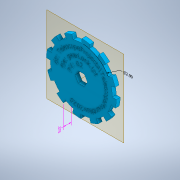
# Autodesk Inventor part: gearLockTopHalf
Saved by Autodesk Inventor 2021.2 (Build 252289000, 289)
## iProperties
Created: 2020-11-07
Part Number: gearLockTopHalf
Material: PC/ABS Plastic
Document SubType Name: Modeling
Designer: robst
Density: 0.357273 g/cm^3
Appearance: Sky Blue Medium
Author: robst
Autodesk Inventor part; units mm, degrees
(part 1 of 2)
ref_plane "YZ Plane" through (0, 0, 0) normal (1, 0, 0) x (0, 1, 0)
ref_plane "XZ Plane" through (0, 0, 0) normal (0, 1, 0) x (-1, 0, 0)
sketch "Sketch1" plane through (0, 0, 0) normal (0, 0, 1) x (1, 0, 0)
  circle A0 centre (0, 0) radius 37.9095
  dimension "d0" = 75.819
  constraints: 1 centre point, 1 coincident
  measures "d0" diameter of A0
extrude "Extrusion1" add sketch "Sketch1" along normal mid plane 9.525
sketch "Sketch10" plane through (0, 0, 4.7625) normal (0, 0, 1) x (1, 0, 0)
  line L0 (7.5523, 0) -> (3.7762, -6.5405)
  line L1 (3.7762, -6.5405) -> (-3.7762, -6.5405)
  line L2 (-3.7762, -6.5405) -> (-7.5523, 0)
  line L3 (-7.5523, 0) -> (-3.7762, 6.5405)
  line L4 (-3.7762, 6.5405) -> (3.7762, 6.5405)
  line L5 (3.7762, 6.5405) -> (7.5523, 0)
  point P0 (0, 0)
  point P1 (0, 0)
  dimension "d55" = 13.081
  constraints: 12 end point, 1 coincident, 1 horizontal, 13 other
  measures "d55" distance between parallel lines of L1 L4
extrude "Extrusion11" cut sketch "Sketch10" against normal through all
sketch "Sketch17" plane through (0, 0, 4.7625) normal (0, 0, 1) x (1, 0, 0)
  circle A0 centre (0, 0) radius 37.9095 projected
  arc A1 (9.4918, 36.702) -> (0, 37.9095) centre (0, 0) ccw
  arc A2 (10.6984, 41.5413) -> (0, 42.8968) centre (0, 0) ccw
  line L0 (0, 0) -> (0, 42.8968) construction
  line L1 (0, 0) -> (0.7487, 42.8902)
  line L2 (9.4918, 36.702) -> (10.6984, 41.5413)
  point P0 (0.6616, 37.9037)
  dimension "d123" = 4.9873
  dimension "d124" = 1
  dimension "d125" = 13
  dimension "d131" = 75.819
  dimension "d132" = 85.7936
  constraints: 6 end point, 5 point on circle, 2 centre point, 2 coincident, 1 concentric, 1 point on line, 1 vertical
  measures "d123" radial gap between concentric circles of A2 A0
  measures "d124" angle of L1 L0
  measures "d125" angle of L2 L1
  measures "d131" diameter of A0
  measures "d132" diameter of A2
extrude "Extrusion19" add sketch "Sketch17" against normal blind 9.525 contours A0 L1 A2 L2
pattern_circular "Circular Pattern11" count 12 over 360 about axis through (0, 0, -10) along (0, 0, 1) of "Extrusion19"
sketch "Sketch28" plane through (0, 0, 4.7625) normal (0, 0, 1) x (1, 0, 0)
  circle A0 centre (0, 0) radius 28.575 construction
  line L0 (-28.4112, 3.3885) -> (-28.4545, 2.7478)
  line L1 (-28.4545, 2.7478) -> (-28.8406, 2.7739)
  spline S0 degree 2 poles (-28.8406, 2.7739) (-28.7274, 2.6177) (-28.5778, 2.3889) (-28.5179, 2.2363) knots 0 0 0 1 2 2 2
  spline S1 degree 2 poles (-28.5179, 2.2363) (-28.4614, 2.0963) (-28.4113, 1.8) (-28.4243, 1.607) knots 0 0 0 1 2 2 2
  spline S2 degree 2 poles (-28.4243, 1.607) (-28.4454, 1.2948) (-28.7397, 0.7866) (-29.0027, 0.6187) knots 0 0 0 1 2 2 2
  spline S3 degree 2 poles (-29.0027, 0.6187) (-29.2657, 0.4508) (-30.0189, 0.2953) (-30.4995, 0.3278) knots 0 0 0 1 2 2 2
  spline S4 degree 2 poles (-30.4995, 0.3278) (-31.0006, 0.3617) (-31.7142, 0.6698) (-31.9741, 0.9143) knots 0 0 0 1 2 2 2
  spline S5 degree 2 poles (-31.9741, 0.9143) (-32.2064, 1.1404) (-32.4501, 1.7469) (-32.4282, 2.0714) knots 0 0 0 1 2 2 2
  spline S6 degree 2 poles (-32.4282, 2.0714) (-32.4091, 2.3548) (-32.2532, 2.7693) (-32.1059, 2.9945) knots 0 0 0 1 2 2 2
  line L2 (-32.1059, 2.9945) -> (-33.7488, 3.1055)
  line L3 (-33.7488, 3.1055) -> (-33.7055, 3.7463)
  line L4 (-33.7055, 3.7463) -> (-28.4112, 3.3885)
  line L5 (-29.3786, 2.8102) -> (-31.5761, 2.9587)
  spline S7 degree 2 poles (-31.5761, 2.9587) (-31.7072, 2.7283) (-31.8189, 2.3562) (-31.8337, 2.1385) knots 0 0 0 1 2 2 2
  spline S8 degree 2 poles (-31.8337, 2.1385) (-31.867, 1.6456) (-31.1654, 1.0371) (-30.4671, 0.9899) knots 0 0 0 1 2 2 2
  spline S9 degree 2 poles (-30.4671, 0.9899) (-29.7935, 0.9444) (-29.0541, 1.3236) (-29.0222, 1.7959) knots 0 0 0 1 2 2 2
  spline S10 degree 2 poles (-29.0222, 1.7959) (-29.0053, 2.0464) (-29.2009, 2.5713) (-29.3786, 2.8102) knots 0 0 0 1 2 2 2
  line L6 (-28.1448, 4.9503) -> (-28.2489, 4.3166)
  line L7 (-28.2489, 4.3166) -> (-32.0105, 4.9348)
  line L8 (-32.0105, 4.9348) -> (-31.9064, 5.5685)
  line L9 (-31.9064, 5.5685) -> (-28.1448, 4.9503)
  line L10 (-32.5246, 5.7159) -> (-32.6428, 4.9969)
  line L11 (-32.6428, 4.9969) -> (-33.3008, 5.1051)
  line L12 (-33.3008, 5.1051) -> (-33.1827, 5.8241)
  line L13 (-33.1827, 5.8241) -> (-32.5246, 5.7159)
  line L14 (-30.5438, 8.57) -> (-30.5514, 8.538)
  spline S11 degree 2 poles (-30.5514, 8.538) (-30.5887, 8.4707) (-30.6341, 8.3165) (-30.6599, 8.2084) knots 0 0 0 1 2 2 2
  spline S12 degree 2 poles (-30.6599, 8.2084) (-30.7203, 7.9562) (-30.6189, 7.407) (-30.4563, 7.1311) knots 0 0 0 1 2 2 2
  line L15 (-30.4563, 7.1311) -> (-27.8259, 6.5017)
  line L16 (-27.8259, 6.5017) -> (-27.9754, 5.8771)
  line L17 (-27.9754, 5.8771) -> (-31.6828, 6.7642)
  line L18 (-31.6828, 6.7642) -> (-31.5333, 7.3888)
  line L19 (-31.5333, 7.3888) -> (-30.9808, 7.2566)
  spline S13 degree 2 poles (-30.9808, 7.2566) (-31.2037, 7.6697) (-31.3302, 8.2376) (-31.2727, 8.4778) knots 0 0 0 1 2 2 2
  spline S14 degree 2 poles (-31.2727, 8.4778) (-31.2497, 8.5739) (-31.2187, 8.6681) (-31.1924, 8.7252) knots 0 0 0 1 2 2 2
  line L20 (-31.1924, 8.7252) -> (-30.5438, 8.57)
  line L21 (-26.9763, 9.4327) -> (-27.2343, 8.6595)
  line L22 (-27.2343, 8.6595) -> (-28.1559, 8.9671)
  line L23 (-28.1559, 8.9671) -> (-27.8979, 9.7403)
  line L24 (-27.8979, 9.7403) -> (-26.9763, 9.4327)
  line L25 (-29.6707, 10.332) -> (-29.9288, 9.5588)
  line L26 (-29.9288, 9.5588) -> (-30.8503, 9.8663)
  line L27 (-30.8503, 9.8663) -> (-30.5923, 10.6395)
  line L28 (-30.5923, 10.6395) -> (-29.6707, 10.332)
  line L29 (-25.0649, 13.7258) -> (-28.9674, 15.9239)
  line L30 (-28.9674, 15.9239) -> (-29.8038, 14.4389)
  line L31 (-29.8038, 14.4389) -> (-30.3275, 14.7339)
  line L32 (-30.3275, 14.7339) -> (-28.3233, 18.2921)
  line L33 (-28.3233, 18.2921) -> (-27.7997, 17.9971)
  line L34 (-27.7997, 17.9971) -> (-28.6361, 16.5121)
  line L35 (-28.6361, 16.5121) -> (-24.7336, 14.314)
  line L36 (-24.7336, 14.314) -> (-25.0649, 13.7258)
  spline S15 degree 2 poles (-22.5342, 17.4324) (-23.0862, 16.7041) (-24.5098, 16.5227) (-25.2644, 17.0946) knots 0 0 0 1 2 2 2
  spline S16 degree 2 poles (-25.2644, 17.0946) (-26.0059, 17.6565) (-26.2959, 19.1005) (-25.8209, 19.7272) knots 0 0 0 1 2 2 2
  spline S17 degree 2 poles (-25.8209, 19.7272) (-25.6071, 20.0093) (-25.1123, 20.3213) (-24.8166, 20.3503) knots 0 0 0 1 2 2 2
  spline S18 degree 2 poles (-24.8166, 20.3503) (-24.5184, 20.3826) (-23.8846, 20.176) (-23.5205, 19.9) knots 0 0 0 1 2 2 2
  line L37 (-23.5205, 19.9) -> (-23.2416, 19.6887)
  line L38 (-23.2416, 19.6887) -> (-24.8355, 17.5856)
  spline S19 degree 2 poles (-24.8355, 17.5856) (-24.3072, 17.1853) (-23.3434, 17.2916) (-22.9853, 17.764) knots 0 0 0 1 2 2 2
  spline S20 degree 2 poles (-22.9853, 17.764) (-22.8585, 17.9313) (-22.6878, 18.3133) (-22.6474, 18.4893) knots 0 0 0 1 2 2 2
  spline S21 degree 2 poles (-22.6474, 18.4893) (-22.6086, 18.6769) (-22.5792, 18.9542) (-22.5844, 19.0563) knots 0 0 0 1 2 2 2
  line L39 (-22.5844, 19.0563) -> (-22.5621, 19.0858)
  line L40 (-22.5621, 19.0858) -> (-22.0043, 18.6631)
  spline S22 degree 2 poles (-22.0043, 18.6631) (-22.0354, 18.5472) (-22.1343, 18.1986) (-22.1843, 18.0712) knots 0 0 0 1 2 2 2
  spline S23 degree 2 poles (-22.1843, 18.0712) (-22.2536, 17.8912) (-22.3949, 17.6161) (-22.5342, 17.4324) knots 0 0 0 1 2 2 2
  spline S24 degree 2 poles (-24.01, 19.4859) (-24.2216, 19.636) (-24.5881, 19.7794) (-24.752, 19.7745) knots 0 0 0 1 2 2 2
  spline S25 degree 2 poles (-24.752, 19.7745) (-24.934, 19.7729) (-25.2667, 19.586) (-25.4234, 19.3794) knots 0 0 0 1 2 2 2
  spline S26 degree 2 poles (-25.4234, 19.3794) (-25.5775, 19.1759) (-25.6725, 18.7985) (-25.6439, 18.5909) knots 0 0 0 1 2 2 2
  spline S27 degree 2 poles (-25.6439, 18.5909) (-25.6095, 18.384) (-25.407, 18.0446) (-25.2259, 17.8815) knots 0 0 0 1 2 2 2
  line L41 (-25.2259, 17.8815) -> (-24.01, 19.4859)
  line L42 (-20.8713, 19.5198) -> (-21.3046, 19.0459)
  line L43 (-21.3046, 19.0459) -> (-25.2207, 22.6267)
  line L44 (-25.2207, 22.6267) -> (-24.7873, 23.1007)
  line L45 (-24.7873, 23.1007) -> (-20.8713, 19.5198)
  spline S28 degree 2 poles (-18.9567, 21.2678) (-19.6329, 20.653) (-21.0656, 20.7357) (-21.7026, 21.4362) knots 0 0 0 1 2 2 2
  spline S29 degree 2 poles (-21.7026, 21.4362) (-22.3285, 22.1246) (-22.3489, 23.5973) (-21.7671, 24.1262) knots 0 0 0 1 2 2 2
  spline S30 degree 2 poles (-21.7671, 24.1262) (-21.5052, 24.3644) (-20.9616, 24.5804) (-20.6656, 24.5547) knots 0 0 0 1 2 2 2
  spline S31 degree 2 poles (-20.6656, 24.5547) (-20.3665, 24.5318) (-19.7813, 24.2125) (-19.4739, 23.8744) knots 0 0 0 1 2 2 2
  line L46 (-19.4739, 23.8744) -> (-19.2385, 23.6155)
  line L47 (-19.2385, 23.6155) -> (-21.1909, 21.8403)
  spline S32 degree 2 poles (-21.1909, 21.8403) (-20.745, 21.3499) (-19.778, 21.2777) (-19.3394, 21.6765) knots 0 0 0 1 2 2 2
  spline S33 degree 2 poles (-19.3394, 21.6765) (-19.1841, 21.8178) (-18.9462, 22.162) (-18.8743, 22.3276) knots 0 0 0 1 2 2 2
  spline S34 degree 2 poles (-18.8743, 22.3276) (-18.8017, 22.5049) (-18.722, 22.7721) (-18.7084, 22.8734) knots 0 0 0 1 2 2 2
  line L48 (-18.7084, 22.8734) -> (-18.681, 22.8984)
  line L49 (-18.681, 22.8984) -> (-18.2102, 22.3806)
  spline S35 degree 2 poles (-18.2102, 22.3806) (-18.262, 22.2723) (-18.4231, 21.9477) (-18.4957, 21.8317) knots 0 0 0 1 2 2 2
  spline S36 degree 2 poles (-18.4957, 21.8317) (-18.5967, 21.6675) (-18.7861, 21.4229) (-18.9567, 21.2678) knots 0 0 0 1 2 2 2
  spline S37 degree 2 poles (-20.031, 23.557) (-20.2116, 23.7434) (-20.5456, 23.9516) (-20.7076, 23.9768) knots 0 0 0 1 2 2 2
  spline S38 degree 2 poles (-20.7076, 23.9768) (-20.8868, 24.0086) (-21.2481, 23.8859) (-21.44, 23.7114) knots 0 0 0 1 2 2 2
  spline S39 degree 2 poles (-21.44, 23.7114) (-21.6289, 23.5397) (-21.7914, 23.1861) (-21.8013, 22.9767) knots 0 0 0 1 2 2 2
  spline S40 degree 2 poles (-21.8013, 22.9767) (-21.8055, 22.7671) (-21.6686, 22.3963) (-21.5205, 22.2028) knots 0 0 0 1 2 2 2
  line L50 (-21.5205, 22.2028) -> (-20.031, 23.557)
  spline S41 degree 2 poles (-16.5837, 23.1592) (-16.8954, 22.937) (-17.5546, 22.72) (-17.7992, 22.6872) knots 0 0 0 1 2 2 2
  line L51 (-17.7992, 22.6872) -> (-18.2173, 23.2739)
  line L52 (-18.2173, 23.2739) -> (-18.1905, 23.293)
  spline S42 degree 2 poles (-18.1905, 23.293) (-18.0852, 23.2872) (-17.8134, 23.2888) (-17.6124, 23.3259) knots 0 0 0 1 2 2 2
  spline S43 degree 2 poles (-17.6124, 23.3259) (-17.4362, 23.3554) (-17.0475, 23.4909) (-16.8765, 23.6127) knots 0 0 0 1 2 2 2
  spline S44 degree 2 poles (-16.8765, 23.6127) (-16.7525, 23.7011) (-16.5081, 23.9612) (-16.4745, 24.0559) knots 0 0 0 1 2 2 2
  spline S45 degree 2 poles (-16.4745, 24.0559) (-16.4227, 24.1889) (-16.4383, 24.3952) (-16.5434, 24.5427) knots 0 0 0 1 2 2 2
  spline S46 degree 2 poles (-16.5434, 24.5427) (-16.6748, 24.7271) (-17.0122, 24.7748) (-17.3157, 24.6545) knots 0 0 0 1 2 2 2
  spline S47 degree 2 poles (-17.3157, 24.6545) (-17.433, 24.6063) (-17.8026, 24.444) (-17.9663, 24.3829) knots 0 0 0 1 2 2 2
  spline S48 degree 2 poles (-17.9663, 24.3829) (-18.3958, 24.2336) (-19.0234, 24.4333) (-19.2408, 24.7384) knots 0 0 0 1 2 2 2
  spline S49 degree 2 poles (-19.2408, 24.7384) (-19.5419, 25.1608) (-19.2834, 26.1387) (-18.7604, 26.5114) knots 0 0 0 1 2 2 2
  spline S50 degree 2 poles (-18.7604, 26.5114) (-18.5023, 26.6954) (-17.8885, 26.9407) (-17.6415, 26.9701) knots 0 0 0 1 2 2 2
  line L53 (-17.6415, 26.9701) -> (-17.2425, 26.4103)
  line L54 (-17.2425, 26.4103) -> (-17.2693, 26.3912)
  spline S51 degree 2 poles (-17.2693, 26.3912) (-17.5852, 26.4087) (-18.206, 26.2443) (-18.4575, 26.0651) knots 0 0 0 1 2 2 2
  spline S52 degree 2 poles (-18.4575, 26.0651) (-18.7156, 25.8811) (-18.9157, 25.4099) (-18.7604, 25.192) knots 0 0 0 1 2 2 2
  spline S53 degree 2 poles (-18.7604, 25.192) (-18.6194, 24.9942) (-18.272, 24.9537) (-17.9943, 25.0606) knots 0 0 0 1 2 2 2
  spline S54 degree 2 poles (-17.9943, 25.0606) (-17.8588, 25.1116) (-17.5275, 25.2568) (-17.3437, 25.3322) knots 0 0 0 1 2 2 2
  spline S55 degree 2 poles (-17.3437, 25.3322) (-16.9396, 25.4887) (-16.3067, 25.3383) (-16.0606, 24.993) knots 0 0 0 1 2 2 2
  spline S56 degree 2 poles (-16.0606, 24.993) (-15.9172, 24.7918) (-15.8215, 24.3242) (-15.8825, 24.0835) knots 0 0 0 1 2 2 2
  spline S57 degree 2 poles (-15.8825, 24.0835) (-15.9489, 23.829) (-16.2652, 23.3862) (-16.5837, 23.1592) knots 0 0 0 1 2 2 2
  spline S58 degree 2 poles (-13.5451, 25.0652) (-13.8904, 24.8728) (-14.5804, 24.7664) (-14.9056, 24.8679) knots 0 0 0 1 2 2 2
  spline S59 degree 2 poles (-14.9056, 24.8679) (-15.2288, 24.9658) (-15.82, 25.4941) (-16.0645, 25.9328) knots 0 0 0 1 2 2 2
  spline S60 degree 2 poles (-16.0645, 25.9328) (-16.309, 26.3715) (-16.4319, 27.1419) (-16.3543, 27.4679) knots 0 0 0 1 2 2 2
  spline S61 degree 2 poles (-16.3543, 27.4679) (-16.2788, 27.7974) (-15.8229, 28.3578) (-15.4849, 28.5462) knots 0 0 0 1 2 2 2
  spline S62 degree 2 poles (-15.4849, 28.5462) (-15.2116, 28.6985) (-14.6147, 28.8284) (-14.3608, 28.8379) knots 0 0 0 1 2 2 2
  line L55 (-14.3608, 28.8379) -> (-14.0102, 28.2086)
  line L56 (-14.0102, 28.2086) -> (-14.0425, 28.1905)
  spline S63 degree 2 poles (-14.0425, 28.1905) (-14.1317, 28.2068) (-14.3909, 28.2321) (-14.562, 28.2263) knots 0 0 0 1 2 2 2
  spline S64 degree 2 poles (-14.562, 28.2263) (-14.7127, 28.2177) (-15.0793, 28.1312) (-15.2231, 28.0511) knots 0 0 0 1 2 2 2
  spline S65 degree 2 poles (-15.2231, 28.0511) (-15.6582, 27.8086) (-15.8202, 26.856) (-15.4855, 26.2554) knots 0 0 0 1 2 2 2
  spline S66 degree 2 poles (-15.4855, 26.2554) (-15.1589, 25.6693) (-14.2816, 25.2957) (-13.8285, 25.5482) knots 0 0 0 1 2 2 2
  spline S67 degree 2 poles (-13.8285, 25.5482) (-13.5552, 25.7005) (-13.1851, 26.2036) (-13.0927, 26.486) knots 0 0 0 1 2 2 2
  line L57 (-13.0927, 26.486) -> (-13.0604, 26.504)
  line L58 (-13.0604, 26.504) -> (-12.7097, 25.8747)
  spline S68 degree 2 poles (-12.7097, 25.8747) (-12.7704, 25.7891) (-12.96, 25.5373) (-13.0466, 25.456) knots 0 0 0 1 2 2 2
  spline S69 degree 2 poles (-13.0466, 25.456) (-13.1664, 25.3327) (-13.3689, 25.1633) (-13.5451, 25.0652) knots 0 0 0 1 2 2 2
  spline S70 degree 2 poles (-9.8925, 28.8813) (-9.53, 27.9888) (-9.9932, 26.6677) (-10.7102, 26.3764) knots 0 0 0 1 2 2 2
  spline S71 degree 2 poles (-10.7102, 26.3764) (-11.4463, 26.0775) (-12.6967, 26.7382) (-13.0468, 27.6002) knots 0 0 0 1 2 2 2
  spline S72 degree 2 poles (-13.0468, 27.6002) (-13.4061, 28.4851) (-12.9346, 29.8185) (-12.2252, 30.1067) knots 0 0 0 1 2 2 2
  spline S73 degree 2 poles (-12.2252, 30.1067) (-11.5081, 30.3979) (-10.2534, 29.77) (-9.8925, 28.8813) knots 0 0 0 1 2 2 2
  spline S74 degree 2 poles (-10.5065, 28.6319) (-10.7854, 29.3184) (-11.5561, 29.783) (-12.0176, 29.5956) knots 0 0 0 1 2 2 2
  spline S75 degree 2 poles (-12.0176, 29.5956) (-12.4791, 29.4081) (-12.7115, 28.5362) (-12.4327, 27.8496) knots 0 0 0 1 2 2 2
  spline S76 degree 2 poles (-12.4327, 27.8496) (-12.1616, 27.1822) (-11.3793, 26.7001) (-10.9178, 26.8875) knots 0 0 0 1 2 2 2
  spline S77 degree 2 poles (-10.9178, 26.8875) (-10.4601, 27.0734) (-10.2308, 27.953) (-10.5065, 28.6319) knots 0 0 0 1 2 2 2
  spline S78 degree 2 poles (-5.9537, 30.0486) (-5.7155, 29.1237) (-6.3152, 27.8045) (-6.9889, 27.631) knots 0 0 0 1 2 2 2
  spline S79 degree 2 poles (-6.9889, 27.631) (-7.264, 27.5601) (-7.7194, 27.5789) (-7.9726, 27.654) knots 0 0 0 1 2 2 2
  line L59 (-7.9726, 27.654) -> (-7.5742, 26.1072)
  line L60 (-7.5742, 26.1072) -> (-8.1961, 25.947)
  line L61 (-8.1961, 25.947) -> (-9.497, 30.998)
  line L62 (-9.497, 30.998) -> (-8.8751, 31.1582)
  line L63 (-8.8751, 31.1582) -> (-8.7755, 30.7715)
  spline S80 degree 2 poles (-8.7755, 30.7715) (-8.5987, 31.0423) (-8.1045, 31.4672) (-7.7736, 31.5524) knots 0 0 0 1 2 2 2
  spline S81 degree 2 poles (-7.7736, 31.5524) (-7.1397, 31.7157) (-6.1714, 30.8938) (-5.9537, 30.0486) knots 0 0 0 1 2 2 2
  spline S82 degree 2 poles (-6.5771, 29.8116) (-6.7403, 30.4454) (-7.3227, 31.0394) (-7.7731, 30.9234) knots 0 0 0 1 2 2 2
  spline S83 degree 2 poles (-7.7731, 30.9234) (-8.0363, 30.8556) (-8.47, 30.4931) (-8.642, 30.2532) knots 0 0 0 1 2 2 2
  line L64 (-8.642, 30.2532) -> (-8.102, 28.1563)
  spline S84 degree 2 poles (-8.102, 28.1563) (-7.829, 28.1033) (-7.4596, 28.1049) (-7.2363, 28.1624) knots 0 0 0 1 2 2 2
  spline S85 degree 2 poles (-7.2363, 28.1624) (-6.754, 28.2866) (-6.4025, 29.1338) (-6.5771, 29.8116) knots 0 0 0 1 2 2 2
  spline S86 degree 2 poles (-3.141, 28.3163) (-4.0483, 28.2065) (-5.1686, 29.1035) (-5.2823, 30.0435) knots 0 0 0 1 2 2 2
  spline S87 degree 2 poles (-5.2823, 30.0435) (-5.3941, 30.9672) (-4.558, 32.1796) (-3.7774, 32.274) knots 0 0 0 1 2 2 2
  spline S88 degree 2 poles (-3.7774, 32.274) (-3.4259, 32.3166) (-2.8576, 32.178) (-2.6311, 31.9856) knots 0 0 0 1 2 2 2
  spline S89 degree 2 poles (-2.6311, 31.9856) (-2.4006, 31.7937) (-2.1084, 31.1946) (-2.0535, 30.7409) knots 0 0 0 1 2 2 2
  line L65 (-2.0535, 30.7409) -> (-2.0115, 30.3936)
  line L66 (-2.0115, 30.3936) -> (-4.6312, 30.0767)
  spline S90 degree 2 poles (-4.6312, 30.0767) (-4.5516, 29.4187) (-3.805, 28.7999) (-3.2165, 28.8711) knots 0 0 0 1 2 2 2
  spline S91 degree 2 poles (-3.2165, 28.8711) (-3.008, 28.8963) (-2.6148, 29.0392) (-2.4602, 29.1326) knots 0 0 0 1 2 2 2
  spline S92 degree 2 poles (-2.4602, 29.1326) (-2.2984, 29.2351) (-2.0787, 29.4068) (-2.009, 29.4816) knots 0 0 0 1 2 2 2
  line L67 (-2.009, 29.4816) -> (-1.9722, 29.486)
  line L68 (-1.9722, 29.486) -> (-1.8881, 28.7913)
  spline S93 degree 2 poles (-1.8881, 28.7913) (-1.9931, 28.733) (-2.3124, 28.5616) (-2.4387, 28.509) knots 0 0 0 1 2 2 2
  spline S94 degree 2 poles (-2.4387, 28.509) (-2.6162, 28.4337) (-2.9122, 28.3439) (-3.141, 28.3163) knots 0 0 0 1 2 2 2
  spline S95 degree 2 poles (-2.6915, 30.8048) (-2.7308, 31.0612) (-2.8826, 31.4244) (-3.0001, 31.5387) knots 0 0 0 1 2 2 2
  spline S96 degree 2 poles (-3.0001, 31.5387) (-3.1277, 31.6684) (-3.4934, 31.7776) (-3.7509, 31.7465) knots 0 0 0 1 2 2 2
  spline S97 degree 2 poles (-3.7509, 31.7465) (-4.0042, 31.7158) (-4.3415, 31.5216) (-4.4708, 31.3567) knots 0 0 0 1 2 2 2
  spline S98 degree 2 poles (-4.4708, 31.3567) (-4.5956, 31.1881) (-4.6987, 30.8066) (-4.69, 30.563) knots 0 0 0 1 2 2 2
  line L69 (-4.69, 30.563) -> (-2.6915, 30.8048)
  spline S99 degree 2 poles (2.1582, 32.1015) (2.1545, 31.7721) (1.9132, 31.182) (1.701, 30.9785) knots 0 0 0 1 2 2 2
  spline S100 degree 2 poles (1.701, 30.9785) (1.4346, 30.7221) (0.7195, 30.4625) (0.1761, 30.4686) knots 0 0 0 1 2 2 2
  line L70 (0.1761, 30.4686) -> (-0.3961, 30.475)
  line L71 (-0.3961, 30.475) -> (-0.4173, 28.5815)
  line L72 (-0.4173, 28.5815) -> (-1.0924, 28.589)
  line L73 (-1.0924, 28.589) -> (-1.0355, 33.6687)
  line L74 (-1.0355, 33.6687) -> (0.2406, 33.6544)
  spline S101 degree 2 poles (0.2406, 33.6544) (0.6934, 33.6494) (1.3256, 33.4941) (1.5666, 33.3226) knots 0 0 0 1 2 2 2
  spline S102 degree 2 poles (1.5666, 33.3226) (1.8485, 33.1259) (2.1629, 32.5255) (2.1582, 32.1015) knots 0 0 0 1 2 2 2
  spline S103 degree 2 poles (1.454, 32.0888) (1.457, 32.3522) (1.2802, 32.7412) (1.0963, 32.8667) knots 0 0 0 1 2 2 2
  spline S104 degree 2 poles (1.0963, 32.8667) (0.937, 32.9756) (0.5098, 33.0668) (0.1929, 33.0703) knots 0 0 0 1 2 2 2
  line L75 (0.1929, 33.0703) -> (-0.367, 33.0766)
  line L76 (-0.367, 33.0766) -> (-0.3896, 31.0513)
  line L77 (-0.3896, 31.0513) -> (0.0714, 31.0462)
  spline S105 degree 2 poles (0.0714, 31.0462) (0.4831, 31.0416) (0.9908, 31.1676) (1.1574, 31.3387) knots 0 0 0 1 2 2 2
  spline S106 degree 2 poles (1.1574, 31.3387) (1.3114, 31.4893) (1.4513, 31.8459) (1.454, 32.0888) knots 0 0 0 1 2 2 2
  line L78 (5.093, 31.3118) -> (5.0603, 31.3158)
  spline S107 degree 2 poles (5.0603, 31.3158) (4.9893, 31.3453) (4.8309, 31.3731) (4.7206, 31.3867) knots 0 0 0 1 2 2 2
  spline S108 degree 2 poles (4.7206, 31.3867) (4.4632, 31.4184) (3.9289, 31.2561) (3.6729, 31.0637) knots 0 0 0 1 2 2 2
  line L79 (3.6729, 31.0637) -> (3.3422, 28.3793)
  line L80 (3.3422, 28.3793) -> (2.7049, 28.4578)
  line L81 (2.7049, 28.4578) -> (3.1709, 32.2412)
  line L82 (3.1709, 32.2412) -> (3.8083, 32.1627)
  line L83 (3.8083, 32.1627) -> (3.7388, 31.5989)
  spline S109 degree 2 poles (3.7388, 31.5989) (4.1244, 31.8666) (4.6745, 32.056) (4.9196, 32.0258) knots 0 0 0 1 2 2 2
  spline S110 degree 2 poles (4.9196, 32.0258) (5.0177, 32.0138) (5.1147, 31.9935) (5.1745, 31.9737) knots 0 0 0 1 2 2 2
  line L84 (5.1745, 31.9737) -> (5.093, 31.3118)
  spline S111 degree 2 poles (8.6902, 29.2655) (8.4679, 28.3282) (7.3244, 27.5205) (6.5714, 27.6991) knots 0 0 0 1 2 2 2
  spline S112 degree 2 poles (6.5714, 27.6991) (5.7983, 27.8825) (5.1629, 29.1459) (5.3776, 30.0512) knots 0 0 0 1 2 2 2
  spline S113 degree 2 poles (5.3776, 30.0512) (5.598, 30.9805) (6.7554, 31.7933) (7.5005, 31.6166) knots 0 0 0 1 2 2 2
  spline S114 degree 2 poles (7.5005, 31.6166) (8.2535, 31.438) (8.9116, 30.1988) (8.6902, 29.2655) knots 0 0 0 1 2 2 2
  spline S115 degree 2 poles (8.0453, 29.4185) (8.2163, 30.1395) (7.8578, 30.9649) (7.3732, 31.0798) knots 0 0 0 1 2 2 2
  spline S116 degree 2 poles (7.3732, 31.0798) (6.8885, 31.1948) (6.1935, 30.6192) (6.0225, 29.8982) knots 0 0 0 1 2 2 2
  spline S117 degree 2 poles (6.0225, 29.8982) (5.8563, 29.1972) (6.214, 28.3508) (6.6987, 28.2359) knots 0 0 0 1 2 2 2
  spline S118 degree 2 poles (6.6987, 28.2359) (7.1793, 28.1219) (7.8762, 28.7055) (8.0453, 29.4185) knots 0 0 0 1 2 2 2
  spline S119 degree 2 poles (9.8099, 26.7294) (9.5969, 26.1148) (8.7119, 25.6982) (8.1324, 25.899) knots 0 0 0 1 2 2 2
  spline S120 degree 2 poles (8.1324, 25.899) (8.0312, 25.934) (7.789, 26.0397) (7.6752, 26.101) knots 0 0 0 1 2 2 2
  line L85 (7.6752, 26.101) -> (7.8638, 26.6456)
  line L86 (7.8638, 26.6456) -> (7.8988, 26.6334)
  spline S121 degree 2 poles (7.8988, 26.6334) (7.9635, 26.5936) (8.1238, 26.5032) (8.2016, 26.4762) knots 0 0 0 1 2 2 2
  spline S122 degree 2 poles (8.2016, 26.4762) (8.4428, 26.3927) (8.7997, 26.4041) (8.9181, 26.5069) knots 0 0 0 1 2 2 2
  spline S123 degree 2 poles (8.9181, 26.5069) (9.0324, 26.5979) (9.2017, 26.9357) (9.2893, 27.1886) knots 0 0 0 1 2 2 2
  line L87 (9.2893, 27.1886) -> (10.3122, 30.141)
  line L88 (10.3122, 30.141) -> (9.6626, 30.366)
  line L89 (9.6626, 30.366) -> (9.8365, 30.8678)
  line L90 (9.8365, 30.8678) -> (11.0929, 30.4325)
  line L91 (11.0929, 30.4325) -> (9.8099, 26.7294)
  line L92 (11.3043, 31.0302) -> (10.6158, 31.2688)
  line L93 (10.6158, 31.2688) -> (10.8342, 31.8989)
  line L94 (10.8342, 31.8989) -> (11.5227, 31.6604)
  line L95 (11.5227, 31.6604) -> (11.3043, 31.0302)
  spline S124 degree 2 poles (12.1886, 25.751) (11.3587, 26.1338) (10.8759, 27.4854) (11.2725, 28.3451) knots 0 0 0 1 2 2 2
  spline S125 degree 2 poles (11.2725, 28.3451) (11.6622, 29.19) (13.0103, 29.7831) (13.7243, 29.4538) knots 0 0 0 1 2 2 2
  spline S126 degree 2 poles (13.7243, 29.4538) (14.0457, 29.3055) (14.4567, 28.8893) (14.5485, 28.6067) knots 0 0 0 1 2 2 2
  spline S127 degree 2 poles (14.5485, 28.6067) (14.644, 28.3223) (14.5783, 27.659) (14.3869, 27.2441) knots 0 0 0 1 2 2 2
  line L96 (14.3869, 27.2441) -> (14.2404, 26.9263)
  line L97 (14.2404, 26.9263) -> (11.8442, 28.0316)
  spline S128 degree 2 poles (11.8442, 28.0316) (11.5666, 27.4297) (11.8773, 26.5112) (12.4156, 26.2629) knots 0 0 0 1 2 2 2
  spline S129 degree 2 poles (12.4156, 26.2629) (12.6062, 26.1749) (13.016, 26.0902) (13.1965, 26.0885) knots 0 0 0 1 2 2 2
  spline S130 degree 2 poles (13.1965, 26.0885) (13.388, 26.0909) (13.6652, 26.1217) (13.7638, 26.1487) knots 0 0 0 1 2 2 2
  line L98 (13.7638, 26.1487) -> (13.7975, 26.1332)
  line L99 (13.7975, 26.1332) -> (13.5043, 25.4977)
  spline S131 degree 2 poles (13.5043, 25.4977) (13.3844, 25.5032) (13.0227, 25.5249) (12.8876, 25.5465) knots 0 0 0 1 2 2 2
  spline S132 degree 2 poles (12.8876, 25.5465) (12.6969, 25.5755) (12.3979, 25.6545) (12.1886, 25.751) knots 0 0 0 1 2 2 2
  spline S133 degree 2 poles (13.8773, 27.6333) (13.9785, 27.8722) (14.0399, 28.2609) (13.9999, 28.4199) knots 0 0 0 1 2 2 2
  spline S134 degree 2 poles (13.9999, 28.4199) (13.9594, 28.5973) (13.7054, 28.8822) (13.4699, 28.9908) knots 0 0 0 1 2 2 2
  spline S135 degree 2 poles (13.4699, 28.9908) (13.2381, 29.0977) (12.8491, 29.1094) (12.6525, 29.0369) knots 0 0 0 1 2 2 2
  spline S136 degree 2 poles (12.6525, 29.0369) (12.4578, 28.959) (12.1698, 28.6884) (12.0494, 28.4764) knots 0 0 0 1 2 2 2
  line L100 (12.0494, 28.4764) -> (13.8773, 27.6333)
  spline S137 degree 2 poles (15.2712, 24.0525) (14.9348, 24.26) (14.5053, 24.8104) (14.4352, 25.1438) knots 0 0 0 1 2 2 2
  spline S138 degree 2 poles (14.4352, 25.1438) (14.3631, 25.4737) (14.5357, 26.2476) (14.7994, 26.675) knots 0 0 0 1 2 2 2
  spline S139 degree 2 poles (14.7994, 26.675) (15.0631, 27.1025) (15.6756, 27.5856) (15.998, 27.677) knots 0 0 0 1 2 2 2
  spline S140 degree 2 poles (15.998, 27.677) (16.3225, 27.7718) (17.0341, 27.6472) (17.3634, 27.4441) knots 0 0 0 1 2 2 2
  spline S141 degree 2 poles (17.3634, 27.4441) (17.6297, 27.2798) (18.0343, 26.8222) (18.1665, 26.6052) knots 0 0 0 1 2 2 2
  line L101 (18.1665, 26.6052) -> (17.7882, 25.9921)
  line L102 (17.7882, 25.9921) -> (17.7567, 26.0115)
  spline S142 degree 2 poles (17.7567, 26.0115) (17.7274, 26.0973) (17.623, 26.3359) (17.5344, 26.4824) knots 0 0 0 1 2 2 2
  spline S143 degree 2 poles (17.5344, 26.4824) (17.4534, 26.6098) (17.1991, 26.8876) (17.059, 26.974) knots 0 0 0 1 2 2 2
  spline S144 degree 2 poles (17.059, 26.974) (16.635, 27.2356) (15.7245, 26.9121) (15.3635, 26.327) knots 0 0 0 1 2 2 2
  spline S145 degree 2 poles (15.3635, 26.327) (15.0112, 25.7559) (15.1132, 24.8079) (15.5546, 24.5355) knots 0 0 0 1 2 2 2
  spline S146 degree 2 poles (15.5546, 24.5355) (15.8209, 24.3712) (16.4406, 24.2937) (16.7322, 24.3508) knots 0 0 0 1 2 2 2
  line L103 (16.7322, 24.3508) -> (16.7637, 24.3314)
  line L104 (16.7637, 24.3314) -> (16.3854, 23.7182)
  spline S147 degree 2 poles (16.3854, 23.7182) (16.2811, 23.7294) (15.9688, 23.7721) (15.8556, 23.8081) knots 0 0 0 1 2 2 2
  spline S148 degree 2 poles (15.8556, 23.8081) (15.6895, 23.8525) (15.4428, 23.9466) (15.2712, 24.0525) knots 0 0 0 1 2 2 2
  spline S149 degree 2 poles (17.6055, 22.4176) (17.1893, 22.734) (17.0819, 23.5655) (17.473, 24.08) knots 0 0 0 1 2 2 2
  line L105 (17.473, 24.08) -> (18.7511, 25.7613)
  line L106 (18.7511, 25.7613) -> (18.4069, 26.0228)
  line L107 (18.4069, 26.0228) -> (18.7283, 26.4456)
  line L108 (18.7283, 26.4456) -> (19.0724, 26.184)
  line L109 (19.0724, 26.184) -> (19.7351, 27.0558)
  line L110 (19.7351, 27.0558) -> (20.2464, 26.6671)
  line L111 (20.2464, 26.6671) -> (19.5837, 25.7954)
  line L112 (19.5837, 25.7954) -> (20.5243, 25.0803)
  line L113 (20.5243, 25.0803) -> (20.2029, 24.6576)
  line L114 (20.2029, 24.6576) -> (19.2623, 25.3726)
  line L115 (19.2623, 25.3726) -> (18.1636, 23.9273)
  spline S150 degree 2 poles (18.1636, 23.9273) (17.9892, 23.6979) (17.8138, 23.4331) (17.7873, 23.2826) knots 0 0 0 1 2 2 2
  spline S151 degree 2 poles (17.7873, 23.2826) (17.7609, 23.1527) (17.8951, 22.9007) (18.0721, 22.7662) knots 0 0 0 1 2 2 2
  spline S152 degree 2 poles (18.0721, 22.7662) (18.1966, 22.6715) (18.4866, 22.57) (18.5565, 22.5531) knots 0 0 0 1 2 2 2
  line L116 (18.5565, 22.5531) -> (18.586, 22.5307)
  line L117 (18.586, 22.5307) -> (18.2372, 22.0718)
  spline S153 degree 2 poles (18.2372, 22.0718) (18.0631, 22.1421) (17.7333, 22.3205) (17.6055, 22.4176) knots 0 0 0 1 2 2 2
  spline S154 degree 2 poles (19.2723, 20.9748) (18.991, 21.2345) (18.6436, 21.8353) (18.5614, 22.068) knots 0 0 0 1 2 2 2
  line L118 (18.5614, 22.068) -> (19.05, 22.5974)
  line L119 (19.05, 22.5974) -> (19.0742, 22.575)
  spline S155 degree 2 poles (19.0742, 22.575) (19.0901, 22.4708) (19.1473, 22.2051) (19.2248, 22.0159) knots 0 0 0 1 2 2 2
  spline S156 degree 2 poles (19.2248, 22.0159) (19.2897, 21.8495) (19.502, 21.4968) (19.6563, 21.3544) knots 0 0 0 1 2 2 2
  spline S157 degree 2 poles (19.6563, 21.3544) (19.7682, 21.2511) (20.0728, 21.0652) (20.1724, 21.0517) knots 0 0 0 1 2 2 2
  spline S158 degree 2 poles (20.1724, 21.0517) (20.3132, 21.0282) (20.5119, 21.0857) (20.6347, 21.2188) knots 0 0 0 1 2 2 2
  spline S159 degree 2 poles (20.6347, 21.2188) (20.7883, 21.3852) (20.7659, 21.7251) (20.586, 21.9976) knots 0 0 0 1 2 2 2
  spline S160 degree 2 poles (20.586, 21.9976) (20.5148, 22.1025) (20.2803, 22.4311) (20.1869, 22.5788) knots 0 0 0 1 2 2 2
  spline S161 degree 2 poles (20.1869, 22.5788) (19.9528, 22.9686) (20.0198, 23.6238) (20.2739, 23.8991) knots 0 0 0 1 2 2 2
  spline S162 degree 2 poles (20.2739, 23.8991) (20.6257, 24.2803) (21.6358, 24.2275) (22.1077, 23.7919) knots 0 0 0 1 2 2 2
  spline S163 degree 2 poles (22.1077, 23.7919) (22.3407, 23.577) (22.7065, 23.0264) (22.7858, 22.7907) knots 0 0 0 1 2 2 2
  line L120 (22.7858, 22.7907) -> (22.3196, 22.2855)
  line L121 (22.3196, 22.2855) -> (22.2954, 22.3079)
  spline S164 degree 2 poles (22.2954, 22.3079) (22.2479, 22.6206) (21.9598, 23.1946) (21.7329, 23.404) knots 0 0 0 1 2 2 2
  spline S165 degree 2 poles (21.7329, 23.404) (21.5, 23.619) (20.9978, 23.7183) (20.8163, 23.5217) knots 0 0 0 1 2 2 2
  spline S166 degree 2 poles (20.8163, 23.5217) (20.6516, 23.3432) (20.683, 22.9949) (20.8445, 22.745) knots 0 0 0 1 2 2 2
  spline S167 degree 2 poles (20.8445, 22.745) (20.9222, 22.6228) (21.1321, 22.3283) (21.2436, 22.1638) knots 0 0 0 1 2 2 2
  spline S168 degree 2 poles (21.2436, 22.1638) (21.4796, 21.8003) (21.4619, 21.15) (21.1743, 20.8384) knots 0 0 0 1 2 2 2
  spline S169 degree 2 poles (21.1743, 20.8384) (21.0068, 20.6569) (20.5687, 20.4674) (20.3206, 20.4779) knots 0 0 0 1 2 2 2
  spline S170 degree 2 poles (20.3206, 20.4779) (20.0579, 20.4907) (19.5597, 20.7096) (19.2723, 20.9748) knots 0 0 0 1 2 2 2
  line L122 (21.5078, 17.1489) -> (21.126, 17.5806)
  line L123 (21.126, 17.5806) -> (24.6094, 23.3168)
  line L124 (24.6094, 23.3168) -> (24.9967, 22.8789)
  line L125 (24.9967, 22.8789) -> (21.5078, 17.1489)
  line L126 (23.2889, 16.5612) -> (26.9698, 19.1131)
  line L127 (26.9698, 19.1131) -> (25.9988, 20.5137)
  line L128 (25.9988, 20.5137) -> (26.4928, 20.8561)
  line L129 (26.4928, 20.8561) -> (28.8195, 17.5)
  line L130 (28.8195, 17.5) -> (28.3255, 17.1576)
  line L131 (28.3255, 17.1576) -> (27.3545, 18.5582)
  line L132 (27.3545, 18.5582) -> (23.6736, 16.0064)
  line L133 (23.6736, 16.0064) -> (23.2889, 16.5612)
  spline S171 degree 2 poles (25.5194, 12.6665) (25.105, 13.481) (25.5631, 14.8411) (26.407, 15.2704) knots 0 0 0 1 2 2 2
  spline S172 degree 2 poles (26.407, 15.2704) (27.2362, 15.6923) (28.662, 15.323) (29.0185, 14.6222) knots 0 0 0 1 2 2 2
  spline S173 degree 2 poles (29.0185, 14.6222) (29.179, 14.3066) (29.2439, 13.7253) (29.1409, 13.4466) knots 0 0 0 1 2 2 2
  spline S174 degree 2 poles (29.1409, 13.4466) (29.0397, 13.1642) (28.5773, 12.6841) (28.17, 12.4769) knots 0 0 0 1 2 2 2
  line L134 (28.17, 12.4769) -> (27.8581, 12.3182)
  line L135 (27.8581, 12.3182) -> (26.6616, 14.6702)
  spline S175 degree 2 poles (26.6616, 14.6702) (26.0709, 14.3696) (25.7458, 13.456) (26.0146, 12.9277) knots 0 0 0 1 2 2 2
  spline S176 degree 2 poles (26.0146, 12.9277) (26.1098, 12.7406) (26.379, 12.4202) (26.5197, 12.3071) knots 0 0 0 1 2 2 2
  spline S177 degree 2 poles (26.5197, 12.3071) (26.6715, 12.1903) (26.9082, 12.0428) (27.0024, 12.003) knots 0 0 0 1 2 2 2
  line L136 (27.0024, 12.003) -> (27.0192, 11.97)
  line L137 (27.0192, 11.97) -> (26.3954, 11.6526)
  spline S178 degree 2 poles (26.3954, 11.6526) (26.3047, 11.7312) (26.0342, 11.9723) (25.9414, 12.0729) knots 0 0 0 1 2 2 2
  spline S179 degree 2 poles (25.9414, 12.0729) (25.8097, 12.2138) (25.6239, 12.461) (25.5194, 12.6665) knots 0 0 0 1 2 2 2
  spline S180 degree 2 poles (28.011, 13.0981) (28.2384, 13.223) (28.5275, 13.4902) (28.5945, 13.6398) knots 0 0 0 1 2 2 2
  spline S181 degree 2 poles (28.5945, 13.6398) (28.6726, 13.8042) (28.6497, 14.1851) (28.5321, 14.4163) knots 0 0 0 1 2 2 2
  spline S182 degree 2 poles (28.5321, 14.4163) (28.4163, 14.6437) (28.1182, 14.8939) (27.9189, 14.9588) knots 0 0 0 1 2 2 2
  spline S183 degree 2 poles (27.9189, 14.9588) (27.7178, 15.0181) (27.324, 14.9841) (27.0982, 14.8923) knots 0 0 0 1 2 2 2
  line L138 (27.0982, 14.8923) -> (28.011, 13.0981)
  line L139 (26.6717, 10.2593) -> (26.4344, 10.8561)
  line L140 (26.4344, 10.8561) -> (31.3654, 12.8166)
  line L141 (31.3654, 12.8166) -> (31.6027, 12.2199)
  line L142 (31.6027, 12.2199) -> (26.6717, 10.2593)
  spline S184 degree 2 poles (27.4089, 7.7738) (27.1508, 8.6505) (27.8505, 9.9035) (28.7588, 10.1709) knots 0 0 0 1 2 2 2
  spline S185 degree 2 poles (28.7588, 10.1709) (29.6513, 10.4336) (30.9852, 9.8092) (31.2072, 9.0549) knots 0 0 0 1 2 2 2
  spline S186 degree 2 poles (31.2072, 9.0549) (31.3072, 8.7152) (31.2643, 8.1319) (31.112, 7.8768) knots 0 0 0 1 2 2 2
  spline S187 degree 2 poles (31.112, 7.8768) (30.9608, 7.6177) (30.4182, 7.2305) (29.9798, 7.1015) knots 0 0 0 1 2 2 2
  line L143 (29.9798, 7.1015) -> (29.6442, 7.0027)
  line L144 (29.6442, 7.0027) -> (28.899, 9.5341)
  spline S188 degree 2 poles (28.899, 9.5341) (28.2632, 9.347) (27.7762, 8.5084) (27.9436, 7.9397) knots 0 0 0 1 2 2 2
  spline S189 degree 2 poles (27.9436, 7.9397) (28.0029, 7.7383) (28.2088, 7.3741) (28.3264, 7.2371) knots 0 0 0 1 2 2 2
  spline S190 degree 2 poles (28.3264, 7.2371) (28.4542, 7.0944) (28.6598, 6.9061) (28.7451, 6.8496) knots 0 0 0 1 2 2 2
  line L145 (28.7451, 6.8496) -> (28.7556, 6.8141)
  line L146 (28.7556, 6.8141) -> (28.0842, 6.6165)
  spline S191 degree 2 poles (28.0842, 6.6165) (28.0094, 6.7103) (27.7877, 6.997) (27.715, 7.1129) knots 0 0 0 1 2 2 2
  spline S192 degree 2 poles (27.715, 7.1129) (27.6113, 7.2755) (27.474, 7.5526) (27.4089, 7.7738) knots 0 0 0 1 2 2 2
  spline S193 degree 2 poles (29.9374, 7.7413) (30.1839, 7.8224) (30.517, 8.0321) (30.6104, 8.1668) knots 0 0 0 1 2 2 2
  spline S194 degree 2 poles (30.6104, 8.1668) (30.7172, 8.3141) (30.7645, 8.6928) (30.6913, 8.9416) knots 0 0 0 1 2 2 2
  spline S195 degree 2 poles (30.6913, 8.9416) (30.6192, 9.1865) (30.372, 9.487) (30.1879, 9.5874) knots 0 0 0 1 2 2 2
  spline S196 degree 2 poles (30.1879, 9.5874) (30.0011, 9.6826) (29.6078, 9.7213) (29.369, 9.6724) knots 0 0 0 1 2 2 2
  line L147 (29.369, 9.6724) -> (29.9374, 7.7413)
  spline S197 degree 2 poles (28.0749, 4.8132) (28.0111, 5.1907) (28.1035, 5.8785) (28.1807, 6.1129) knots 0 0 0 1 2 2 2
  line L148 (28.1807, 6.1129) -> (28.8911, 6.233)
  line L149 (28.8911, 6.233) -> (28.8966, 6.2005)
  spline S198 degree 2 poles (28.8966, 6.2005) (28.8454, 6.1084) (28.7282, 5.8631) (28.6738, 5.666) knots 0 0 0 1 2 2 2
  spline S199 degree 2 poles (28.6738, 5.666) (28.6235, 5.4947) (28.5757, 5.0858) (28.6108, 4.8788) knots 0 0 0 1 2 2 2
  spline S200 degree 2 poles (28.6108, 4.8788) (28.6362, 4.7286) (28.7635, 4.3952) (28.8341, 4.3237) knots 0 0 0 1 2 2 2
  spline S201 degree 2 poles (28.8341, 4.3237) (28.9311, 4.219) (29.1235, 4.143) (29.3021, 4.1732) knots 0 0 0 1 2 2 2
  spline S202 degree 2 poles (29.3021, 4.1732) (29.5253, 4.211) (29.7155, 4.4936) (29.7398, 4.8192) knots 0 0 0 1 2 2 2
  spline S203 degree 2 poles (29.7398, 4.8192) (29.7476, 4.9458) (29.7629, 5.3492) (29.7794, 5.5232) knots 0 0 0 1 2 2 2
  spline S204 degree 2 poles (29.7794, 5.5232) (29.8324, 5.9747) (30.2861, 6.4522) (30.6554, 6.5147) knots 0 0 0 1 2 2 2
  spline S205 degree 2 poles (30.6554, 6.5147) (31.1669, 6.6012) (31.9339, 5.9419) (32.041, 5.3086) knots 0 0 0 1 2 2 2
  spline S206 degree 2 poles (32.041, 5.3086) (32.0939, 4.9961) (32.0467, 4.3368) (31.9654, 4.1018) knots 0 0 0 1 2 2 2
  line L150 (31.9654, 4.1018) -> (31.2875, 3.9871)
  line L151 (31.2875, 3.9871) -> (31.2821, 4.0196)
  spline S207 degree 2 poles (31.2821, 4.0196) (31.4357, 4.2961) (31.5587, 4.9265) (31.5072, 5.2309) knots 0 0 0 1 2 2 2
  spline S208 degree 2 poles (31.5072, 5.2309) (31.4544, 5.5434) (31.1177, 5.9291) (30.8539, 5.8844) knots 0 0 0 1 2 2 2
  spline S209 degree 2 poles (30.8539, 5.8844) (30.6144, 5.8439) (30.4263, 5.5491) (30.4013, 5.2526) knots 0 0 0 1 2 2 2
  spline S210 degree 2 poles (30.4013, 5.2526) (30.3881, 5.1084) (30.3741, 4.747) (30.3617, 4.5486) knots 0 0 0 1 2 2 2
  spline S211 degree 2 poles (30.3617, 4.5486) (30.3262, 4.1168) (29.9146, 3.6129) (29.4965, 3.5422) knots 0 0 0 1 2 2 2
  spline S212 degree 2 poles (29.4965, 3.5422) (29.2529, 3.501) (28.7904, 3.619) (28.6005, 3.779) knots 0 0 0 1 2 2 2
  spline S213 degree 2 poles (28.6005, 3.779) (28.4005, 3.9497) (28.1401, 4.4276) (28.0749, 4.8132) knots 0 0 0 1 2 2 2
  spline S214 degree 2 poles (28.4636, 1.2475) (28.4412, 1.6421) (28.6466, 2.3094) (28.8799, 2.5576) knots 0 0 0 1 2 2 2
  spline S215 degree 2 poles (28.8799, 2.5576) (29.1091, 2.8057) (29.8424, 3.1071) (30.3438, 3.1356) knots 0 0 0 1 2 2 2
  spline S216 degree 2 poles (30.3438, 3.1356) (30.8452, 3.1641) (31.592, 2.9385) (31.8515, 2.7264) knots 0 0 0 1 2 2 2
  spline S217 degree 2 poles (31.8515, 2.7264) (32.115, 2.5146) (32.4202, 1.8598) (32.4422, 1.4735) knots 0 0 0 1 2 2 2
  spline S218 degree 2 poles (32.4422, 1.4735) (32.4599, 1.1611) (32.3163, 0.5674) (32.2141, 0.3349) knots 0 0 0 1 2 2 2
  line L152 (32.2141, 0.3349) -> (31.4948, 0.294)
  line L153 (31.4948, 0.294) -> (31.4927, 0.331)
  spline S219 degree 2 poles (31.4927, 0.331) (31.5463, 0.4041) (31.6821, 0.6263) (31.7516, 0.7828) knots 0 0 0 1 2 2 2
  spline S220 degree 2 poles (31.7516, 0.7828) (31.8096, 0.9221) (31.8918, 1.2897) (31.8825, 1.4541) knots 0 0 0 1 2 2 2
  spline S221 degree 2 poles (31.8825, 1.4541) (31.8542, 1.9514) (31.0678, 2.5128) (30.3814, 2.4739) knots 0 0 0 1 2 2 2
  spline S222 degree 2 poles (30.3814, 2.4739) (29.7115, 2.4358) (28.9925, 1.8095) (29.0219, 1.2916) knots 0 0 0 1 2 2 2
  spline S223 degree 2 poles (29.0219, 1.2916) (29.0396, 0.9792) (29.3308, 0.4267) (29.5445, 0.2203) knots 0 0 0 1 2 2 2
  line L154 (29.5445, 0.2203) -> (29.5466, 0.1834)
  line L155 (29.5466, 0.1834) -> (28.8274, 0.1425)
  spline S224 degree 2 poles (28.8274, 0.1425) (28.7768, 0.2345) (28.633, 0.5149) (28.5977, 0.6284) knots 0 0 0 1 2 2 2
  spline S225 degree 2 poles (28.5977, 0.6284) (28.5391, 0.79) (28.475, 1.0461) (28.4636, 1.2475) knots 0 0 0 1 2 2 2
  spline S226 degree 2 poles (30.3029, -3.7044) (29.3417, -3.641) (28.3552, -2.6477) (28.4061, -1.8755) knots 0 0 0 1 2 2 2
  spline S227 degree 2 poles (28.4061, -1.8755) (28.4584, -1.0827) (29.5986, -0.2461) (30.527, -0.3073) knots 0 0 0 1 2 2 2
  spline S228 degree 2 poles (30.527, -0.3073) (31.48, -0.3702) (32.4739, -1.3764) (32.4235, -2.1404) knots 0 0 0 1 2 2 2
  spline S229 degree 2 poles (32.4235, -2.1404) (32.3726, -2.9127) (31.26, -3.7676) (30.3029, -3.7044) knots 0 0 0 1 2 2 2
  spline S230 degree 2 poles (30.3466, -3.0431) (31.086, -3.0919) (31.8403, -2.6011) (31.8731, -2.1041) knots 0 0 0 1 2 2 2
  spline S231 degree 2 poles (31.8731, -2.1041) (31.9059, -1.6071) (31.2228, -1.0174) (30.4834, -0.9687) knots 0 0 0 1 2 2 2
  spline S232 degree 2 poles (30.4834, -0.9687) (29.7645, -0.9213) (28.9893, -1.4147) (28.9566, -1.9118) knots 0 0 0 1 2 2 2
  spline S233 degree 2 poles (28.9566, -1.9118) (28.9241, -2.4047) (29.6154, -2.9949) (30.3466, -3.0431) knots 0 0 0 1 2 2 2
  spline S234 degree 2 poles (29.6342, -7.7577) (28.6981, -7.5684) (27.7728, -6.4531) (27.9108, -5.7712) knots 0 0 0 1 2 2 2
  spline S235 degree 2 poles (27.9108, -5.7712) (27.9671, -5.4927) (28.1827, -5.0911) (28.3607, -4.8961) knots 0 0 0 1 2 2 2
  line L156 (28.3607, -4.8961) -> (26.7952, -4.5795)
  line L157 (26.7952, -4.5795) -> (26.9225, -3.95)
  line L158 (26.9225, -3.95) -> (32.0348, -4.984)
  line L159 (32.0348, -4.984) -> (31.9075, -5.6135)
  line L160 (31.9075, -5.6135) -> (31.5161, -5.5343)
  spline S236 degree 2 poles (31.5161, -5.5343) (31.6826, -5.8116) (31.8492, -6.4417) (31.7814, -6.7766) knots 0 0 0 1 2 2 2
  spline S237 degree 2 poles (31.7814, -6.7766) (31.6517, -7.4182) (30.4896, -7.9308) (29.6342, -7.7577) knots 0 0 0 1 2 2 2
  spline S238 degree 2 poles (29.6929, -7.0934) (30.3345, -7.2232) (31.1231, -6.9585) (31.2153, -6.5025) knots 0 0 0 1 2 2 2
  spline S239 degree 2 poles (31.2153, -6.5025) (31.2691, -6.2362) (31.1323, -5.6877) (30.9915, -5.4283) knots 0 0 0 1 2 2 2
  line L161 (30.9915, -5.4283) -> (28.8691, -4.999)
  spline S240 degree 2 poles (28.8691, -4.999) (28.7023, -5.2214) (28.5426, -5.5545) (28.4969, -5.7805) knots 0 0 0 1 2 2 2
  spline S241 degree 2 poles (28.4969, -5.7805) (28.3981, -6.2687) (29.007, -6.9547) (29.6929, -7.0934) knots 0 0 0 1 2 2 2
  spline S242 degree 2 poles (26.8479, -9.5323) (27.1452, -8.6681) (28.4412, -8.0516) (29.3366, -8.3596) knots 0 0 0 1 2 2 2
  spline S243 degree 2 poles (29.3366, -8.3596) (30.2164, -8.6622) (30.9423, -9.9436) (30.6866, -10.6871) knots 0 0 0 1 2 2 2
  spline S244 degree 2 poles (30.6866, -10.6871) (30.5714, -11.0219) (30.1987, -11.4727) (29.9268, -11.5925) knots 0 0 0 1 2 2 2
  spline S245 degree 2 poles (29.9268, -11.5925) (29.6535, -11.7162) (28.987, -11.7177) (28.5548, -11.5691) knots 0 0 0 1 2 2 2
  line L162 (28.5548, -11.5691) -> (28.224, -11.4552)
  line L163 (28.224, -11.4552) -> (29.0822, -8.9599)
  spline S246 degree 2 poles (29.0822, -8.9599) (28.4554, -8.7443) (27.5729, -9.146) (27.3801, -9.7066) knots 0 0 0 1 2 2 2
  spline S247 degree 2 poles (27.3801, -9.7066) (27.3118, -9.9051) (27.2688, -10.3213) (27.2853, -10.5012) knots 0 0 0 1 2 2 2
  spline S248 degree 2 poles (27.2853, -10.5012) (27.3069, -10.6914) (27.3655, -10.9641) (27.4023, -11.0595) knots 0 0 0 1 2 2 2
  line L164 (27.4023, -11.0595) -> (27.3903, -11.0945)
  line L165 (27.3903, -11.0945) -> (26.7285, -10.8669)
  spline S249 degree 2 poles (26.7285, -10.8669) (26.7218, -10.7471) (26.707, -10.385) (26.7148, -10.2484) knots 0 0 0 1 2 2 2
  spline S250 degree 2 poles (26.7148, -10.2484) (26.7245, -10.0558) (26.773, -9.7503) (26.8479, -9.5323) knots 0 0 0 1 2 2 2
  spline S251 degree 2 poles (28.8907, -11.0229) (29.1386, -11.0994) (29.5316, -11.1214) (29.6858, -11.0656) knots 0 0 0 1 2 2 2
  spline S252 degree 2 poles (29.6858, -11.0656) (29.8582, -11.0073) (30.116, -10.726) (30.2004, -10.4807) knots 0 0 0 1 2 2 2
  spline S253 degree 2 poles (30.2004, -10.4807) (30.2834, -10.2394) (30.2558, -9.8511) (30.1639, -9.6628) knots 0 0 0 1 2 2 2
  spline S254 degree 2 poles (30.1639, -9.6628) (30.0667, -9.477) (29.7684, -9.2177) (29.5454, -9.1192) knots 0 0 0 1 2 2 2
  line L166 (29.5454, -9.1192) -> (28.8907, -11.0229)
  line L167 (24.1963, -15.3562) -> (24.5137, -14.7603)
  line L168 (24.5137, -14.7603) -> (28.376, -16.8177)
  line L169 (28.376, -16.8177) -> (26.3722, -14.2484)
  line L170 (26.3722, -14.2484) -> (26.5658, -13.8851)
  line L171 (26.5658, -13.8851) -> (29.8101, -14.1253)
  line L172 (29.8101, -14.1253) -> (25.9478, -12.068)
  line L173 (25.9478, -12.068) -> (26.2439, -11.5121)
  line L174 (26.2439, -11.5121) -> (30.7275, -13.9004)
  line L175 (30.7275, -13.9004) -> (30.294, -14.7143)
  line L176 (30.294, -14.7143) -> (27.2018, -14.5037)
  line L177 (27.2018, -14.5037) -> (29.1211, -16.9161)
  line L178 (29.1211, -16.9161) -> (28.6799, -17.7445)
  line L179 (28.6799, -17.7445) -> (24.1963, -15.3562)
  spline S255 degree 2 poles (23.2425, -19.7933) (22.4755, -19.2106) (22.1998, -17.838) (22.668, -17.2217) knots 0 0 0 1 2 2 2
  spline S256 degree 2 poles (22.668, -17.2217) (23.1486, -16.5891) (24.561, -16.5195) (25.3019, -17.0823) knots 0 0 0 1 2 2 2
  spline S257 degree 2 poles (25.3019, -17.0823) (26.0624, -17.66) (26.3372, -19.0474) (25.874, -19.6571) knots 0 0 0 1 2 2 2
  spline S258 degree 2 poles (25.874, -19.6571) (25.4058, -20.2734) (24.0063, -20.3735) (23.2425, -19.7933) knots 0 0 0 1 2 2 2
  spline S259 degree 2 poles (23.6435, -19.2655) (24.2335, -19.7138) (25.1334, -19.7201) (25.4347, -19.3234) knots 0 0 0 1 2 2 2
  spline S260 degree 2 poles (25.4347, -19.3234) (25.736, -18.9268) (25.4911, -18.0583) (24.901, -17.6101) knots 0 0 0 1 2 2 2
  spline S261 degree 2 poles (24.901, -17.6101) (24.3273, -17.1743) (23.4085, -17.1588) (23.1072, -17.5554) knots 0 0 0 1 2 2 2
  spline S262 degree 2 poles (23.1072, -17.5554) (22.8084, -17.9488) (23.0599, -18.8223) (23.6435, -19.2655) knots 0 0 0 1 2 2 2
  line L180 (19.1891, -21.2251) -> (19.6425, -20.7703)
  line L181 (19.6425, -20.7703) -> (19.9399, -21.0668)
  spline S263 degree 2 poles (19.9399, -21.0668) (19.9655, -20.6738) (20.151, -20.1088) (20.3835, -19.8756) knots 0 0 0 1 2 2 2
  spline S264 degree 2 poles (20.3835, -19.8756) (20.5579, -19.7007) (20.9855, -19.505) (21.2242, -19.5163) knots 0 0 0 1 2 2 2
  spline S265 degree 2 poles (21.2242, -19.5163) (21.4659, -19.5247) (21.9756, -19.7772) (22.2497, -20.0504) knots 0 0 0 1 2 2 2
  line L182 (22.2497, -20.0504) -> (24.0017, -21.7973)
  line L183 (24.0017, -21.7973) -> (23.5483, -22.252)
  line L184 (23.5483, -22.252) -> (22.0091, -20.7173)
  spline S266 degree 2 poles (22.0091, -20.7173) (21.7933, -20.5022) (21.4786, -20.2524) (21.3184, -20.2031) knots 0 0 0 1 2 2 2
  spline S267 degree 2 poles (21.3184, -20.2031) (21.1582, -20.1539) (20.8731, -20.2474) (20.6958, -20.4253) knots 0 0 0 1 2 2 2
  spline S268 degree 2 poles (20.6958, -20.4253) (20.5301, -20.5914) (20.3446, -21.1564) (20.3247, -21.4505) knots 0 0 0 1 2 2 2
  line L185 (20.3247, -21.4505) -> (22.3421, -23.4619)
  line L186 (22.3421, -23.4619) -> (21.8886, -23.9166)
  line L187 (21.8886, -23.9166) -> (19.1891, -21.2251)
  line L188 (16.1095, -23.6495) -> (16.6204, -23.2604)
  line L189 (16.6204, -23.2604) -> (17.9372, -24.9898)
  spline S269 degree 2 poles (17.9372, -24.9898) (18.0968, -25.1994) (18.4105, -25.5297) (18.5517, -25.5929) knots 0 0 0 1 2 2 2
  spline S270 degree 2 poles (18.5517, -25.5929) (18.7013, -25.6602) (19.0088, -25.6019) (19.1987, -25.4573) knots 0 0 0 1 2 2 2
  spline S271 degree 2 poles (19.1987, -25.4573) (19.3887, -25.3126) (19.6369, -24.8028) (19.7055, -24.4919) knots 0 0 0 1 2 2 2
  line L190 (19.7055, -24.4919) -> (17.9796, -22.2254)
  line L191 (17.9796, -22.2254) -> (18.4906, -21.8364)
  line L192 (18.4906, -21.8364) -> (20.8, -24.8692)
  line L193 (20.8, -24.8692) -> (20.2891, -25.2583)
  line L194 (20.2891, -25.2583) -> (20.0322, -24.9209)
  spline S272 degree 2 poles (20.0322, -24.9209) (19.96, -25.3019) (19.6825, -25.8547) (19.4336, -26.0443) knots 0 0 0 1 2 2 2
  spline S273 degree 2 poles (19.4336, -26.0443) (18.9881, -26.3834) (18.0348, -26.178) (17.6084, -25.6179) knots 0 0 0 1 2 2 2
  line L195 (17.6084, -25.6179) -> (16.1095, -23.6495)
  spline S274 degree 2 poles (14.3147, -24.6494) (14.7626, -24.3798) (15.5748, -24.5876) (15.9081, -25.1413) knots 0 0 0 1 2 2 2
  line L196 (15.9081, -25.1413) -> (16.9973, -26.9506)
  line L197 (16.9973, -26.9506) -> (17.3676, -26.7277)
  line L198 (17.3676, -26.7277) -> (17.6415, -27.1827)
  line L199 (17.6415, -27.1827) -> (17.2712, -27.4056)
  line L200 (17.2712, -27.4056) -> (17.836, -28.3438)
  line L201 (17.836, -28.3438) -> (17.2857, -28.675)
  line L202 (17.2857, -28.675) -> (16.721, -27.7368)
  line L203 (16.721, -27.7368) -> (15.7088, -28.3462)
  line L204 (15.7088, -28.3462) -> (15.4349, -27.8912)
  line L205 (15.4349, -27.8912) -> (16.4471, -27.2818)
  line L206 (16.4471, -27.2818) -> (15.5108, -25.7264)
  spline S275 degree 2 poles (15.5108, -25.7264) (15.3622, -25.4796) (15.1811, -25.2186) (15.051, -25.1383) knots 0 0 0 1 2 2 2
  spline S276 degree 2 poles (15.051, -25.1383) (14.9401, -25.0657) (14.6563, -25.0972) (14.4659, -25.2119) knots 0 0 0 1 2 2 2
  spline S277 degree 2 poles (14.4659, -25.2119) (14.3318, -25.2926) (14.1303, -25.5244) (14.0887, -25.5831) knots 0 0 0 1 2 2 2
  line L207 (14.0887, -25.5831) -> (14.0569, -25.6022)
  line L208 (14.0569, -25.6022) -> (13.7597, -25.1084)
  spline S278 degree 2 poles (13.7597, -25.1084) (13.8894, -24.9727) (14.1771, -24.7322) (14.3147, -24.6494) knots 0 0 0 1 2 2 2
  line L209 (9.9801, -26.8371) -> (10.6718, -26.5286)
  line L210 (10.6718, -26.5286) -> (14.5089, -29.6133)
  line L211 (14.5089, -29.6133) -> (12.7246, -25.613)
  line L212 (12.7246, -25.613) -> (13.2999, -25.3564)
  line L213 (13.2999, -25.3564) -> (15.3692, -29.9958)
  line L214 (15.3692, -29.9958) -> (14.4932, -30.3866)
  line L215 (14.4932, -30.3866) -> (10.9863, -27.5468)
  line L216 (10.9863, -27.5468) -> (12.6246, -31.22)
  line L217 (12.6246, -31.22) -> (12.0494, -31.4766)
  line L218 (12.0494, -31.4766) -> (9.9801, -26.8371)
  spline S279 degree 2 poles (6.5454, -29.8186) (6.2867, -28.8907) (6.8971, -27.6307) (7.6426, -27.4229) knots 0 0 0 1 2 2 2
  spline S280 degree 2 poles (7.6426, -27.4229) (8.4079, -27.2096) (9.575, -28.0082) (9.8249, -28.9044) knots 0 0 0 1 2 2 2
  spline S281 degree 2 poles (9.8249, -28.9044) (10.0814, -29.8244) (9.4613, -31.0955) (8.7237, -31.3012) knots 0 0 0 1 2 2 2
  spline S282 degree 2 poles (8.7237, -31.3012) (7.9782, -31.509) (6.803, -30.7425) (6.5454, -29.8186) knots 0 0 0 1 2 2 2
  spline S283 degree 2 poles (7.1839, -29.6406) (7.3829, -30.3544) (8.0958, -30.9035) (8.5756, -30.7698) knots 0 0 0 1 2 2 2
  spline S284 degree 2 poles (8.5756, -30.7698) (9.0554, -30.636) (9.3854, -29.7961) (9.1864, -29.0823) knots 0 0 0 1 2 2 2
  spline S285 degree 2 poles (9.1864, -29.0823) (8.993, -28.3884) (8.2706, -27.8205) (7.7907, -27.9543) knots 0 0 0 1 2 2 2
  spline S286 degree 2 poles (7.7907, -27.9543) (7.3149, -28.0869) (6.9871, -28.9348) (7.1839, -29.6406) knots 0 0 0 1 2 2 2
  line L219 (2.9735, -32.296) -> (3.8451, -28.3165)
  line L220 (3.8451, -28.3165) -> (4.4154, -28.2333)
  line L221 (4.4154, -28.2333) -> (6.375, -31.7999)
  line L222 (6.375, -31.7999) -> (5.6866, -31.9003)